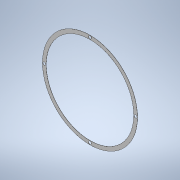
# Autodesk Inventor part: cage_electrode
Saved by Autodesk Inventor 2021 (Build 250183000, 183)
## iProperties
Created: 2020-07-14
Part Number: cage_electrode
Material: Generic
Document SubType Name: Modeling
Designer: aydan
Density: 1 g/cm^3
Appearance: Default
Author: aydan
Autodesk Inventor part; units mm, degrees
ref_plane "YZ Plane" through (0, 0, 0) normal (1, 0, 0) x (0, 1, 0)
ref_plane "XZ Plane" through (0, 0, 0) normal (0, 1, 0) x (-1, 0, 0)
ref_plane "XY Plane" through (0, 0, 0) normal (0, 0, 1) x (1, 0, 0)
sketch "Sketch1" plane through (0, 0, 0) normal (0, 0, 1) x (1, 0, 0)
  circle A0 centre (0, 0) radius 30
  circle A1 centre (0, 0) radius 32.5
  dimension "d0" = 60
  dimension "d1" = 2.5
  constraints: 2 centre point, 1 coincident
  measures "d0" diameter of A0
  measures "d1" radial gap between concentric circles of A0 A1
extrude "Extrusion1" add sketch "Sketch1" along normal blind 0.1
sketch "Sketch2" plane through (0, 0, 0.1) normal (0, 0, 1) x (1, 0, 0)
  circle A0 centre (0, 31.25) radius 1
  circle A1 centre (0, 0) radius 32.5 projected
  circle A2 centre (31.25, 0) radius 1
  circle A3 centre (-31.25, 0) radius 1
  circle A4 centre (-0.0425, -31.25) radius 1
  dimension "d4" = 2
  dimension "d5" = 0.25
  dimension "d6" = 2
  dimension "d7" = 0.25
  dimension "d8" = 2
  dimension "d9" = 0.25
  dimension "d10" = 2
  dimension "d11" = 0.25
  constraints: 4 centre point
  measures "d4" diameter of A0
  measures "d6" diameter of A2
  measures "d8" diameter of A3
  measures "d10" diameter of A4
extrude "Extrusion2" cut sketch "Sketch2" against normal blind 0.2 contours A0 | A2 | A3 | A4
body "Solid1"
